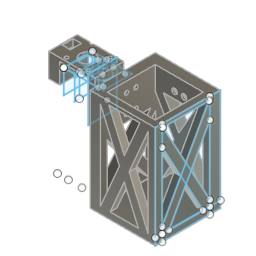
Chocolate_Extruder_v12_v4 (Autodesk Fusion 360 design; units mm, degrees)
Autodesk Fusion 360 part; units mm, degrees
note: some values were not read from the file. Chosen so that the rebuilt part matches the saved one: which pieces of a blend or face edit are solid. Set by a fixed rule: which sketch regions a step uses.
sketch "Sketch1" plane through (0, 0, 0) normal (0, 0, 1) x (1, 0, 0)
  line L0 (0, 70.5) -> (70.5, 70.5)
  line L1 (70.5, 70.5) -> (70.5, 0)
  line L2 (70.5, 0) -> (0, 0)
  line L3 (0, 0) -> (0, 70.5)
  line L4 (-15, 85.5) -> (75.5, 85.5)
  line L5 (75.5, 85.5) -> (75.5, -5)
  line L6 (75.5, -5) -> (-15, -5)
  line L7 (-15, -5) -> (-15, 85.5)
  circle A0 centre (35.25, 35.25) radius 5.5
  dimension "d1" = 70.5
  dimension "d2" = 70.5
  dimension "d3" = 5
  dimension "d4" = 5
  dimension "d5" = 15
  dimension "d6" = 15
  dimension "d9" = 11
  dimension "d10" = 35.25
  dimension "d11" = 35.25
  constraint horizontal L0
  constraint vertical L1
  constraint horizontal L2
  constraint vertical L3
  constraint coincident L2.end L3.start
  constraint horizontal L4
  constraint vertical L5
  constraint horizontal L6
  constraint vertical L7
  measures "d1" distance of L1 L3
  measures "d2" distance of L0 L2
  measures "d3" distance of L1 L5
  measures "d4" distance of L2 L6
  measures "d5" distance of L0 L4
  measures "d6" distance of L3 L7
  measures "d9" diameter of A0
  measures "d10" distance of L3 A0.centre
  measures "d11" distance of L0 A0.centre
extrude "Extrude1" add sketch "Sketch1" along normal blind 140 contours L4 L5 L6 L7 makes body 1
extrude "Extrude2" add sketch "Sketch1" against normal blind 10 contours L0 L1 L2 L3 | L4 L5 L6 L7 bodies 1
sketch "Sketch2" plane through (0, 0, -10) normal (0, 0, -1) x (1, 0, 0)
  circle A0 centre (35.25, -35.25) radius 5.5
  line L0 (75.5, 5) -> (-15, 5)
  line L1 (-15, 5) -> (-15, -85.5)
  line L2 (-15, -85.5) -> (75.5, -85.5)
  line L3 (75.5, -85.5) -> (75.5, 5)
ref_plane "WorkPlane1" through (35.25, 35.25, 125) normal (0, 0, -1) x (1, 0, 0)
sketch "Sketch3" plane through (0, 0, 125) normal (0, 0, -1) x (-1, 0, 0)
  line L0 (15, 14.25) -> (57, 14.25)
  line L1 (57, 14.25) -> (57, 56.25)
  line L2 (57, 56.25) -> (15, 56.25)
  line L3 (15, 56.25) -> (15, 14.25)
  circle A0 centre (36, 34.25) radius 11
  circle A1 centre (36, 34.25) radius 16
  circle A2 centre (20, 19.25) radius 2.5
  circle A3 centre (20, 51.25) radius 2.2361
  line L4 (15, -5) -> (15, 85.5)
  circle A4 centre (52, 19.25) radius 2.5
  circle A5 centre (52, 51.25) radius 2.2361
  dimension "d15" = 21
  dimension "d16" = 20
  dimension "d17" = 22
  dimension "d18" = 42
  dimension "d19" = 22
  dimension "d20" = 5
  dimension "d21" = 5
  dimension "d22" = 5
  dimension "d23" = 5
  dimension "d24" = 5
  dimension "d26" = 42
  dimension "d27" = 19.25
  dimension "d28" = 29.25
  dimension "d29" = 5
  dimension "d30" = 5
  constraint horizontal L0
  constraint vertical L1
  constraint vertical L3
  constraint coincident L2.end L4
  measures "d15" distance of L3 A0.centre
  measures "d16" distance of L0 A0.centre
  measures "d17" distance of L2 A0.centre
  measures "d18" distance of L0 L2
  measures "d19" diameter of A0
  measures "d21" distance of L0 A2.centre
  measures "d22" distance of L3 A2.centre
  measures "d23" diameter of A2
  measures "d24" distance of L3 A3.centre
  measures "d26" distance of L1 L3
  measures "d27" distance of L0 L4.start
  measures "d28" distance of L2.end L4.end
  measures "d29" diameter of A4
  measures "d30" distance of L0 A4.centre
extrude "Extrude3" add sketch "Sketch3" against normal blind 5 separate body contours L0 L1 L2 L3 L4 | A1 makes body 2
sketch "Sketch4" plane through (0, 0, 130) normal (0, 0, 1) x (-1, 0, 0)
  circle A0 centre (36, -34.25) radius 11
  circle A1 centre (20, -51.25) radius 2.2361
  circle A2 centre (20, -19.25) radius 2.5
  circle A3 centre (52, -19.25) radius 2.5
  line L0 (15, -14.25) -> (15, -56.25)
  line L1 (15, -56.25) -> (57, -56.25)
  line L2 (57, -56.25) -> (57, -14.25)
  circle A4 centre (36, -34.25) radius 6
  line L3 (36, -34.25) -> (57, -34.25)
  line L4 (36, -34.25) -> (15, -34.25)
  circle A5 centre (52, -51.25) radius 2.2361
  dimension "d36" = 12
  constraint concentric A0 A4
  constraint coincident A0.centre A4.centre
  constraint coincident L2 L3.end
  constraint perpendicular L2 L3
  constraint coincident L0 L4.end
  constraint perpendicular L0 L4
  measures "d36" diameter of A4
ref_plane "WorkPlane2" through (-36, 34.25, 127.5) normal (0, -1, 0) x (1, 0, 0)
sketch "Sketch5" plane through (0, 34.25, 0) normal (0, -1, 0) x (-1, 0, 0)
  line L0 (30, -130) -> (42, -130)
  line L1 (42, -130) -> (42, -150)
  line L2 (42, -150) -> (30, -150)
  line L3 (30, -150) -> (30, -130)
  line L4 (42.8404, -129.1596) -> (42.8404, -150.8404)
  line L5 (42.8404, -150.8404) -> (29.1596, -150.8404)
  line L6 (29.1596, -150.8404) -> (29.1596, -129.1596)
  line L7 (29.1596, -129.1596) -> (42.8404, -129.1596)
  line L8 (30, -130) -> (29.1596, -130)
  line L9 (29.1596, -130) -> (42, -130)
  line L10 (42.8404, -130) -> (42, -130)
  line L11 (52.8404, -130) -> (42.8404, -140)
  line L12 (36, -130) -> (57, -130)
  line L13 (29.1596, -140) -> (19.1596, -130)
  line L14 (36, -130) -> (15, -130)
  line L15 (24.1596, -130) -> (29.1596, -135)
  line L16 (47.8404, -130) -> (42.8404, -135)
  line L17 (36, -150) -> (36, -150.8404)
  line L18 (42.8404, -135) -> (42, -135.8404)
  line L19 (29.1596, -135) -> (30, -135.8404)
  line L20 (42, -150) -> (42.8404, -150)
  point P0 (36, -130)
  point P1 (36, -150)
  dimension "d38" = 6
  dimension "d39" = 6
  dimension "d40" = -0.8404
  dimension "d41" = 20
  dimension "d42" = 10
  dimension "d43" = 10
  dimension "d44" = 10
  dimension "d45" = 10
  dimension "d46" = 5
  dimension "d47" = 5
  dimension "d48" = 5
  dimension "d49" = 5
  constraint horizontal L0
  constraint vertical L1
  constraint horizontal L2
  constraint vertical L3
  constraint coincident L0 P0
  constraint coincident L6 L8.end
  constraint perpendicular L6 L8
  constraint coincident L4 L10.start
  constraint perpendicular L1 L10
  constraint coincident L4 L11.end
  constraint coincident L11.start L12
  constraint coincident L6 L13.start
  constraint coincident L13.end L14
  constraint midpoint L2 P1
  constraint coincident L14 L15.start
  constraint coincident L6 L15.end
  constraint coincident L12 L16.start
  constraint coincident L4 L16.end
  constraint coincident P1 L17.start
  constraint midpoint L5 L17.end
  constraint coincident L1 L18.end
  constraint parallel L16 L18
  constraint coincident L3 L19.end
  constraint perpendicular L18 L19
  constraint coincident L4 L20.end
  constraint perpendicular L4 L20
  measures "d38" distance of L1 P0
  measures "d39" distance of L3 P0
  measures "d41" distance of L0 L2
  measures "d42" distance of L10.start L11.end
  measures "d43" distance of L10.start L11.start
  measures "d44" distance of L8.end L13.end
  measures "d45" distance of L8.end L13.start
  measures "d46" distance of L6 L15.start
  measures "d47" distance of L8.end L15.end
  measures "d48" distance of L10.start L16.start
  measures "d49" distance of L10.start L16.end
revolve "Revolve1" [suppressed]
sketch "Sketch6" plane through (-57, 0, 0) normal (-1, 0, 0) x (0, -1, 0)
  line L0 (-56.25, 125) -> (-14.25, 125)
  line L1 (-14.25, 125) -> (-14.25, 130)
  line L2 (-14.25, 130) -> (-56.25, 130)
  line L3 (-56.25, 130) -> (-56.25, 125)
  line L4 (-56.25, 130) -> (-14.25, 130)
  line L5 (-14.25, 130) -> (-14.25, 95)
  line L6 (-14.25, 95) -> (-56.25, 95)
  line L7 (-56.25, 95) -> (-56.25, 130)
  line L8 (-49.25, 130) -> (-49.25, 95)
  line L9 (-21.25, 130) -> (-21.25, 95)
  dimension "d51" = 30
  dimension "d151" = 7
  dimension "d152" = 7
  constraint horizontal L4
  constraint vertical L5
  constraint horizontal L6
  constraint vertical L7
  constraint coincident L2.end L3.start
  constraint coincident L0.end L5
  constraint coincident L4 L8.start
  constraint coincident L6 L8.end
  constraint perpendicular L6 L8
  constraint coincident L4 L9.start
  constraint coincident L6 L9.end
  constraint perpendicular L6 L9
  measures "d51" distance of L0 L6
  measures "d151" distance of L7 L8
  measures "d152" distance of L5 L9
extrude "Extrude4" add sketch "Sketch6" along normal blind 16 bodies 2
sketch "Sketch7" plane through (-73, 0, 0) normal (-1, 0, 0) x (0, -1, 0)
  line L0 (-56.25, 95) -> (-14.25, 95)
  line L1 (-14.25, 130) -> (-56.25, 130)
  line L2 (-14.25, 95) -> (-14.25, 130)
  line L3 (-56.25, 130) -> (-56.25, 95)
sketch "Sketch8" plane through (0, 0, 130) normal (0, 0, 1) x (-1, 0, 0)
  circle A0 centre (20, -51.25) radius 2.2361
  circle A1 centre (52, -19.25) radius 2.5
  circle A2 centre (20, -19.25) radius 2.5
  line L0 (73, -14.25) -> (15, -14.25)
  line L1 (15, -14.25) -> (15, -56.25)
  line L2 (15, -56.25) -> (73, -56.25)
  line L3 (73, -56.25) -> (73, -14.25)
  line L4 (59, -27) -> (71, -27)
  line L5 (71, -27) -> (71, -43)
  line L6 (71, -43) -> (59, -43)
  line L7 (59, -43) -> (59, -27)
  line L8 (73, -14.25) -> (73, -56.25)
  circle A3 centre (36, -34.25) radius 11
  circle A4 centre (52, -51.25) radius 2.2361
  dimension "d54" = 2
  dimension "d55" = 16
  dimension "d56" = 12
  constraint horizontal L4
  constraint vertical L5
  constraint horizontal L6
  constraint vertical L7
  measures "d54" distance of L5 L8
  measures "d55" distance of L4 L6
  measures "d56" distance of L5 L7
extrude "Extrude5" cut sketch "Sketch8" against normal blind 10 contours L4 L5 L6 L7 bodies 2
sketch "Sketch11" plane through (0, 70.5, 0) normal (0, -1, 0) x (1, 0, 0)
  line L0 (0, 0) -> (70.5, 0)
  line L1 (70.5, 0) -> (70.5, 140)
  line L2 (70.5, 140) -> (0, 140)
  line L3 (0, 140) -> (0, 0)
  circle A0 centre (28.25, 120) radius 4
  circle A1 centre (42.25, 120) radius 4
  circle A2 centre (28.25, 120) radius 2
  circle A3 centre (42.25, 120) radius 2
  line L4 (0, 0) -> (70.5, 0)
  dimension "d77" = 8
  dimension "d78" = 28.25
  dimension "d79" = 14
  dimension "d80" = 8
  dimension "d83" = 4
  dimension "d84" = 4
  dimension "d87" = 120
  constraint concentric A0 A2
  constraint concentric A1 A3
  measures "d77" diameter of A0
  measures "d78" distance of L1 A1.centre
  measures "d79" distance of A0.centre A1.centre
  measures "d80" diameter of A1
  measures "d83" diameter of A2
  measures "d84" diameter of A3
  measures "d87" distance of A1.centre L4
extrude "Extrude8" cut sketch "Sketch11" against normal blind 3 contours A0 | A1 | A2 | A3 bodies 1
extrude "Extrude9" cut sketch "Sketch11" against normal blind 15 contours A2 | A3 bodies 1
move_body "Move1" bodies 2 to x (1, 0, 0) y (0, 1, 0) z (0, 0, 1) at (-22.0189, -0.0781, 10)
sketch "Sketch12" plane through (-37.0189, 0, 0) normal (1, 0, 0) x (0, 1, 0)
  line L0 (14.1719, 135) -> (56.1719, 135)
  line L1 (56.1719, 135) -> (56.1719, 140)
  line L2 (56.1719, 140) -> (14.1719, 140)
  line L3 (14.1719, 140) -> (14.1719, 135)
  line L4 (14.1719, 140) -> (56.1719, 140)
  line L5 (56.1719, 140) -> (56.1719, 75)
  line L6 (56.1719, 75) -> (14.1719, 75)
  line L7 (14.1719, 75) -> (14.1719, 140)
  point P0 (51.25, 130)
  dimension "d88" = 42
  dimension "d93" = 60
  constraint horizontal L4
  constraint vertical L5
  constraint horizontal L6
  constraint vertical L7
  constraint coincident L2.end L3.start
  measures "d88" distance of L5 L7
  measures "d93" distance of L0 L6
extrude "Extrude10" add sketch "Sketch12" along normal blind 10 bodies 2
sketch "Sketch16" plane through (0, 0, 0) normal (1, 0, 0) x (0, 1, 0)
  line L0 (0, 0) -> (70.5, 0)
  line L1 (70.5, 0) -> (70.5, 140)
  line L2 (70.5, 140) -> (0, 140)
  line L3 (0, 140) -> (0, 0)
  line L4 (0, 125) -> (70.5, 125)
  line L5 (0, 98) -> (70.5, 98)
  circle A0 centre (28.25, 125) radius 2
  circle A1 centre (42.25, 125) radius 2
  circle A2 centre (28.25, 98) radius 2
  circle A3 centre (42.25, 98) radius 2
  line L6 (70.5, 140) -> (70.5, 0)
  circle A4 centre (42.25, 125) radius 3
  circle A5 centre (28.25, 125) radius 3
  circle A6 centre (28.25, 98) radius 3
  circle A7 centre (42.25, 98) radius 3
  point P0 (35.25, 140)
  dimension "d121" = 4
  dimension "d122" = 4
  dimension "d123" = 4
  dimension "d124" = 4
  dimension "d125" = 14
  dimension "d126" = 14
  dimension "d127" = 28.25
  dimension "d128" = 28.25
  dimension "d129" = 28.25
  dimension "d130" = 28.25
  dimension "d131" = 1
  dimension "d132" = 1
  dimension "d133" = 1
  dimension "d134" = 1
  dimension "d137" = 15
  dimension "d138" = 27
  constraint coincident L3 L4.start
  constraint coincident L1 L4.end
  constraint perpendicular L1 L4
  constraint coincident L3 L5.start
  constraint coincident L1 L5.end
  constraint perpendicular L1 L5
  constraint coincident L4 A0.centre
  constraint coincident L4 A1.centre
  constraint coincident L5 A2.centre
  constraint coincident L5 A3.centre
  constraint midpoint L2 P0
  measures "d121" diameter of A0
  measures "d122" diameter of A1
  measures "d123" diameter of A2
  measures "d124" diameter of A3
  measures "d125" distance of A0.centre A1.centre
  measures "d126" distance of A2.centre A3.centre
  measures "d127" distance of A1.centre L6
  measures "d128" distance of L3 A0.centre
  measures "d129" distance of L3 A2.centre
  measures "d130" distance of A3.centre L6
  measures "d137" distance of L2 L4
  measures "d138" distance of L4 L5
extrude "Extrude14" cut sketch "Sketch16" against normal blind 37.019 contours L5 A2 | L5 A2 | L5 A3 | L5 A3 | L4 A0 | L4 A0 | L4 A1 | L4 A1 bodies 1 2
extrude "Extrude15" cut sketch "Sketch16" against normal blind 3 contours L5 A2 A6 | L5 A2 A6 | L5 A3 A7 | L5 A3 A7 | L4 A0 A5 | L4 A0 A5 | L5 A2 | L5 A2 | L4 A1 A4 | L4 A1 A4 | L5 A3 | L5 A3 | L4 A0 | L4 A0 | L4 A1 | L4 A1 bodies 1
sketch "Sketch21" plane through (75.5, 0, 0) normal (1, 0, 0) x (0, 1, 0)
  line L0 (85.5, -10) -> (85.5, 140)
  line L1 (85.5, 140) -> (-5, 140)
  line L2 (-5, 140) -> (-5, -10)
  line L3 (-5, -10) -> (85.5, -10)
  line L4 (0, 0) -> (0, -10)
  line L5 (0, 0) -> (0, 140)
  line L6 (70, 140) -> (70, -10)
  line L7 (0, 135) -> (70, 135)
  line L8 (0, 0) -> (70, 0)
  line L9 (0, 110) -> (60, 0)
  line L10 (1.1565, 135) -> (70, 8.787)
  line L11 (10, 0) -> (70, 110)
  line L12 (68.5277, 135) -> (0, 9.366)
  line L13 (85.5, 0) -> (-5, 0)
  dimension "d149" = 5
  dimension "d150" = 10
  constraint coincident L4.start L5.start
  constraint coincident L3 L4.end
  constraint perpendicular L3 L4
  constraint coincident L1 L5.end
  constraint perpendicular L1 L5
  constraint coincident L1 L6.start
  constraint coincident L3 L6.end
  constraint perpendicular L3 L6
  constraint coincident L5 L7.start
  constraint coincident L6 L7.end
  constraint perpendicular L6 L7
  constraint coincident L6 L8.end
  constraint perpendicular L6 L8
  constraint coincident L5 L9.start
  constraint coincident L8 L9.end
  constraint coincident L7 L10.start
  constraint coincident L6 L10.end
  constraint parallel L9 L10
  constraint coincident L8 L11.start
  constraint coincident L6 L11.end
  constraint coincident L7 L12.start
  constraint coincident L5 L12.end
  constraint parallel L11 L12
  measures "d149" distance of L1 L7
  measures "d150" distance of L3 L13
extrude "Extrude18" cut sketch "Sketch21" against normal blind 10 contours L6 L10 L11 | L8 L9 L11 L13 | L5 L9 L12 | L7 L10 L12 bodies 1
sketch "Sketch22" plane through (0, -5, 0) normal (0, -1, 0) x (1, 0, 0)
  line L0 (75.5, -10) -> (75.5, 140)
  line L1 (75.5, 140) -> (-15, 140)
  line L2 (-15, 140) -> (-15, -10)
  line L3 (-15, -10) -> (75.5, -10)
  line L4 (0, 140) -> (0, -10)
  line L5 (70, 140) -> (70, -10)
  line L6 (60, -10) -> (0, 130)
  line L7 (10, -10) -> (70, 130)
  line L8 (60, 140) -> (0, 0)
  line L9 (10, 140) -> (70, 0)
  line L10 (-15, 0) -> (75.5, 0)
  line L11 (75.5, 134.8901) -> (-15, 134.8901)
  constraint coincident L1 L4.start
  constraint coincident L3 L4.end
  constraint perpendicular L3 L4
  constraint coincident L1 L5.start
  constraint coincident L3 L5.end
  constraint perpendicular L3 L5
  constraint coincident L3 L6.start
  constraint coincident L4 L6.end
  constraint coincident L3 L7.start
  constraint coincident L5 L7.end
  constraint coincident L1 L8.start
  constraint coincident L8.end origin
  constraint parallel L7 L8
  constraint coincident L1 L9.start
  constraint coincident L5 L9.end
  constraint parallel L6 L9
  constraint coincident L2 L10.start
  constraint coincident L0 L10.end
  constraint perpendicular L0 L10
  constraint coincident L0 L11.start
  constraint coincident L2 L11.end
  constraint perpendicular L2 L11
extrude "Extrude19" cut sketch "Sketch22" against normal blind 10 contours L5 L7 L9 | L6 L7 L10 | L8 L9 L11 | L4 L6 L8 bodies 1
sketch "Sketch23" plane through (0, 85.5, 0) normal (0, 1, 0) x (-1, 0, 0)
  circle A0 centre (-42.25, 120) radius 2
  circle A1 centre (-28.25, 120) radius 2
  line L0 (15, -10) -> (15, 140)
  line L1 (15, 140) -> (-75.5, 140)
  line L2 (-75.5, 140) -> (-75.5, -10)
  line L3 (-75.5, -10) -> (15, -10)
  line L4 (-70, 140) -> (-70, -10)
  line L5 (0, 140) -> (0, -10)
  line L6 (-75.5, 0) -> (15, 0)
  line L7 (-75.5, 110) -> (15, 110)
  line L8 (-70, 110) -> (-10, 0)
  line L9 (0, 10) -> (-57.4408, 110)
  line L10 (-60.3129, 0) -> (0, 105.9676)
  line L11 (-11.909, 110) -> (-70, 7.9362)
  dimension "d155" = 10
  constraint coincident L1 L4.start
  constraint coincident L3 L4.end
  constraint perpendicular L3 L4
  constraint coincident L1 L5.start
  constraint coincident L3 L5.end
  constraint perpendicular L3 L5
  constraint coincident L2 L6.start
  constraint coincident L0 L6.end
  constraint perpendicular L0 L6
  constraint coincident L2 L7.start
  constraint coincident L0 L7.end
  constraint perpendicular L0 L7
  constraint coincident L4 L8.start
  constraint coincident L6 L8.end
  constraint coincident L5 L9.start
  constraint coincident L7 L9.end
  constraint coincident L6 L10.start
  constraint coincident L5 L10.end
  constraint coincident L7 L11.start
  constraint coincident L4 L11.end
  constraint parallel L10 L11
  measures "d155" distance of A0.centre L7
extrude "Extrude20" cut sketch "Sketch23" against normal blind 15 contours L5 L9 L10 | L6 L8 L10 | L7 L9 L11 | L4 L8 L11 bodies 1
sketch "Sketch24" plane through (-15, 0, 0) normal (-1, 0, 0) x (0, -1, 0)
  circle A0 centre (-42.25, 125) radius 2
  circle A1 centre (-42.25, 98) radius 2
  circle A2 centre (-28.25, 125) radius 2
  circle A3 centre (-28.25, 98) radius 2
  line L0 (5, -10) -> (5, 140)
  line L1 (5, 140) -> (-85.5, 140)
  line L2 (-85.5, 140) -> (-85.5, -10)
  line L3 (-85.5, -10) -> (5, -10)
  line L4 (-85.5, 88) -> (5, 88)
  line L5 (-85.5, 0.6227) -> (5, 0.6227)
  line L6 (0.0167, 140) -> (0.0167, -10)
  line L7 (-70.8768, 140) -> (-70.8768, -10)
  line L8 (-70.8768, 80.9133) -> (-9.5001, 0.6227)
  line L9 (-63.7873, 88) -> (0.0167, 10.341)
  line L10 (-61.9234, 0.6227) -> (0.0167, 79.5561)
  line L11 (-9.5001, 88) -> (-70.8768, 9.7847)
  dimension "d158" = 10
  constraint coincident L2 L4.start
  constraint coincident L0 L4.end
  constraint perpendicular L0 L4
  constraint coincident L2 L5.start
  constraint coincident L0 L5.end
  constraint perpendicular L0 L5
  constraint coincident L1 L6.start
  constraint coincident L3 L6.end
  constraint perpendicular L3 L6
  constraint coincident L1 L7.start
  constraint coincident L3 L7.end
  constraint perpendicular L3 L7
  constraint coincident L7 L8.start
  constraint coincident L5 L8.end
  constraint coincident L4 L9.start
  constraint coincident L6 L9.end
  constraint coincident L5 L10.start
  constraint coincident L6 L10.end
  constraint coincident L4 L11.start
  constraint coincident L7 L11.end
  constraint parallel L10 L11
  measures "d158" distance of A3.centre L4
extrude "Extrude21" cut sketch "Sketch24" against normal blind 15 contours L5 L8 L10 | L6 L9 L10 | L4 L9 L11 | L7 L8 L11 bodies 1
copy_body "Body->Comp1" bodies 1 removing the originals makes body 3 in component "Component"
copy_body "Body->Comp2" bodies 2 removing the originals makes body 4 in component "Component'"
fillet "Fillet1" radius 5 48 edges at (57.4408, 78, 110) (11.909, 78, 110) (35, -2.5, 81.6667) (42.1429, -2.5, 65) (27.8571, -2.5, 65) (35, -2.5, 48.3333) (34.5705, 78, 70.1846) (27.4359, 78, 57.7637) (41.5723, 78, 57.8826) (34.6213, 78, 45.1391) (10, 78, 0) (60.3129, 78, 0) (0, 78.1884, 10) (-7.5, 70.8768, 9.7847) (70, 78, 7.9362) (73, 70, 8.787) (73, 60, 0) (73, 10, 0) (70, -2.5, 0) (73, 0, 9.366) (0, -2.5, 0) (14.2857, -2.5, 0) (55.7143, -2.5, 0) (73, 42.3964, 59.3935) (73, 27.4456, 59.683) (73, 34.8421, 73.2431) (73, 35, 45.8333) (73, 1.1565, 135) (73, 68.5277, 135) (12.19, -2.5, 134.8901) (57.81, -2.5, 134.8901) (0, -2.5, 130) (70, -2.5, 130) (73, 70, 110) (73, 0, 110) (70, 78, 110) (0, 78, 105.9676) (-7.5, 61.9234, 0.6227) (-7.5, 9.5001, 0.6227) (-7.5, -0.0167, 10.341) (-7.5, 27.7638, 44.154) (-7.5, 35.3686, 34.4628) (-7.5, 43.3344, 44.8834) (-7.5, 36.0206, 54.2037) (-7.5, 9.5001, 88) (-7.5, 63.7873, 88) (-7.5, -0.0167, 79.5561) (-7.5, 70.8768, 80.9133) on bodies 3 in component "Component"
sketch "Sketch25" plane through (0, 85.5, 0) normal (0, 1, 0) x (-1, 0, 0)
  line L0 (-30.3248, 37.2621) -> (-14.0332, 7.3943)
  arc A0 (-18.4227, 0) -> (-14.0332, 7.3943) centre (-18.4227, 5) ccw
  line L1 (-18.4227, 0) -> (-51.7139, 0)
  arc A1 (-56.0594, 7.4733) -> (-51.7139, 0) centre (-51.7139, 5) ccw
  line L2 (-56.0594, 7.4733) -> (-39.0597, 37.3411)
  arc A2 (-30.3248, 37.2621) -> (-39.0597, 37.3411) centre (-34.7143, 34.8678) ccw
  line L3 (-42.9506, 55.4611) -> (-60.6546, 24.3558)
  arc A3 (-70, 26.8291) -> (-60.6546, 24.3558) centre (-65, 26.8291) ccw
  line L4 (-70, 26.8291) -> (-70, 90.3917)
  arc A4 (-60.6105, 92.786) -> (-70, 90.3917) centre (-65, 90.3917) ccw
  line L5 (-60.6105, 92.786) -> (-42.9065, 60.3287)
  arc A5 (-42.9506, 55.4611) -> (-42.9065, 60.3287) centre (-47.296, 57.9344) ccw
  line L6 (-26.0217, 60.2484) -> (-9.3454, 89.548)
  arc A6 (0, 87.0747) -> (-9.3454, 89.548) centre (-5, 87.0747) ccw
  line L7 (0, 87.0747) -> (0, 28.743)
  arc A7 (-9.3356, 26.2526) -> (0, 28.743) centre (-5, 28.743) ccw
  line L8 (-9.3356, 26.2526) -> (-26.0119, 55.2847)
  arc A8 (-26.0217, 60.2484) -> (-26.0119, 55.2847) centre (-21.6763, 57.7751) ccw
  line L9 (-38.9261, 77.7672) -> (-53.1383, 102.5096)
  arc A9 (-48.8026, 110) -> (-53.1383, 102.5096) centre (-48.8026, 105) ccw
  line L10 (-48.8026, 110) -> (-20.508, 110)
  arc A10 (-16.1626, 102.5267) -> (-20.508, 110) centre (-20.508, 105) ccw
  line L11 (-16.1626, 102.5267) -> (-30.245, 77.7844)
  arc A11 (-38.9261, 77.7672) -> (-30.245, 77.7844) centre (-34.5904, 80.2577) ccw
  circle A12 centre (-42.25, 120) radius 2
  circle A13 centre (-28.25, 120) radius 2
  line L12 (15, -10) -> (15, 140)
  line L13 (15, 140) -> (-75.5, 140)
  line L14 (-75.5, 140) -> (-75.5, -10)
  line L15 (-75.5, -10) -> (15, -10)
  circle A14 centre (-42.25, 120) radius 2
  circle A15 centre (-28.25, 120) radius 2
  line L16 (-42.25, 110) -> (-28.25, 110)
  arc A16 (-28.25, 110) -> (-28.25, 130) centre (-28.25, 120) ccw
  line L17 (-28.25, 130) -> (-42.25, 130)
  arc A17 (-42.25, 130) -> (-42.25, 110) centre (-42.25, 120) ccw
  line L18 (-42.25, 120) -> (-28.25, 120) construction
  dimension "d163" = 20
  constraint tangent L16 A16
  constraint tangent A16 L17
  constraint parallel L16 L17
  constraint tangent L17 A17
  constraint tangent L16 A17
  constraint coincident A13.centre A15.centre
  constraint coincident A12.centre A14.centre
  measures "d163" diameter of A16
extrude "Extrude1'" cut sketch "Sketch25" against normal blind 10 contours L12 L13 L14 L15 bodies 3 in component "Component"
sketch "Sketch1 (2)" plane through (-15, 0, 0) normal (-1, 0, 0) x (0, -1, 0) in component "Component"
  line L0 (-75.5, 140) -> (-75.5, -10)
  line L1 (-75.5, -10) -> (5, -10)
  line L2 (5, -10) -> (5, 140)
  line L3 (5, 140) -> (-75.5, 140)
  circle A0 centre (-28.25, 98) radius 2
  circle A1 centre (-28.25, 125) radius 2
  circle A2 centre (-42.25, 98) radius 2
  circle A3 centre (-42.25, 125) radius 2
  line L4 (-8.8466, 21.1289) -> (-25.215, 41.0518)
  arc A4 (-25.2852, 47.3125) -> (-25.215, 41.0518) centre (-21.3517, 44.2259) ccw
  line L5 (-25.2852, 47.3125) -> (-8.9168, 68.1717)
  arc A5 (0.0167, 65.085) -> (-8.9168, 68.1717) centre (-4.9833, 65.085) ccw
  line L6 (0.0167, 65.085) -> (0.0167, 24.303)
  arc A6 (-8.8466, 21.1289) -> (0.0167, 24.303) centre (-4.9833, 24.303) ccw
  line L7 (-31.448, 29.3341) -> (-15.6435, 8.6593)
  arc A7 (-19.6158, 0.6227) -> (-15.6435, 8.6593) centre (-19.6158, 5.6227) ccw
  line L8 (-19.6158, 0.6227) -> (-51.6441, 0.6227)
  arc A8 (-55.5776, 8.7094) -> (-51.6441, 0.6227) centre (-51.6441, 5.6227) ccw
  line L9 (-55.5776, 8.7094) -> (-39.3538, 29.3842)
  arc A9 (-31.448, 29.3341) -> (-39.3538, 29.3842) centre (-35.4203, 26.2975) ccw
  line L10 (-15.8459, 79.9133) -> (-32.1766, 59.1023)
  arc A10 (-39.9734, 59.0149) -> (-32.1766, 59.1023) centre (-36.1101, 62.189) ccw
  line L11 (-39.9734, 59.0149) -> (-57.0716, 79.8259)
  arc A11 (-53.2082, 88) -> (-57.0716, 79.8259) centre (-53.2082, 83) ccw
  line L12 (-53.2082, 88) -> (-19.7794, 88)
  arc A12 (-15.8459, 79.9133) -> (-19.7794, 88) centre (-19.7794, 83) ccw
  line L13 (-45.7251, 41.8368) -> (-61.9433, 21.1691)
  arc A13 (-70.8768, 24.2557) -> (-61.9433, 21.1691) centre (-65.8768, 24.2557) ccw
  line L14 (-70.8768, 24.2557) -> (-70.8768, 66.1395)
  arc A14 (-61.9045, 69.176) -> (-70.8768, 66.1395) centre (-65.8768, 66.1395) ccw
  line L15 (-61.9045, 69.176) -> (-45.6863, 47.96)
  arc A15 (-45.7251, 41.8368) -> (-45.6863, 47.96) centre (-49.6586, 44.9234) ccw
  circle A16 centre (-28.25, 125) radius 2
  circle A17 centre (-42.25, 125) radius 2
  circle A18 centre (-42.25, 98) radius 2
  circle A19 centre (-28.25, 98) radius 2
  line L16 (-28.25, 125) -> (-42.25, 98) construction
  line L17 (-43.25, 130) -> (-27.25, 130)
  line L18 (-23.25, 126) -> (-23.25, 97)
  line L19 (-27.25, 93) -> (-43.25, 93)
  line L20 (-47.25, 97) -> (-47.25, 126)
  line L21 (-47.25, 130) -> (-23.25, 93) construction
  line L22 (-23.25, 130) -> (-47.25, 93) construction
  arc A20 (-43.25, 130) -> (-47.25, 126) centre (-43.25, 126) ccw
  arc A21 (-47.25, 97) -> (-43.25, 93) centre (-43.25, 97) ccw
  arc A22 (-27.25, 93) -> (-23.25, 97) centre (-27.25, 97) ccw
  arc A23 (-23.25, 126) -> (-27.25, 130) centre (-27.25, 126) ccw
  point P0 (-35.25, 111.5)
  point P1 (-35.25, 111.5)
  dimension "d166" = 5
  dimension "d167" = 5
  dimension "d168" = 4
  dimension "d169" = 4
  constraint coincident A1.centre A16.centre
  constraint coincident A2.centre A18.centre
  constraint midpoint L16 P1
  constraint horizontal L17
  constraint perpendicular L17 L18
  constraint parallel L17 L19
  constraint parallel L18 L20
  constraint coincident L21 P1
  constraint coincident L22 P1
  constraint coincident P1 P0
  constraint coincident L21.start L17
  constraint coincident L21.start L20
  constraint tangent L17 A20
  constraint tangent L20 A20
  constraint coincident L22.end L19
  constraint coincident L22.end L20
  constraint tangent L19 A21
  constraint tangent L20 A21
  constraint equal A20 A21
  constraint coincident L21.end L19
  constraint coincident L21.end L18
  constraint tangent L19 A22
  constraint tangent L18 A22
  constraint equal A20 A22
  constraint coincident L22.start L17
  constraint coincident L22.start L18
  constraint tangent L17 A23
  constraint tangent L18 A23
  measures "d166" distance of A3.centre L17
  measures "d167" distance of A3.centre L20
  measures "d168" radius of A20
  measures "d169" radius of A23
extrude "Extrude2'" cut sketch "Sketch1 (2)" against normal blind 10 contours L0 L1 L2 L3 bodies 3 in component "Component"
extrude "Extrude3'" cut 1 faces at (35.387, 6.5885, -10) along direction (0, 0, 1) blind 5 on bodies 3 bodies 3 in component "Component"
sketch "Sketch1 (3)" plane through (-27.0189, 0, 0) normal (1, 0, 0) x (0, 1, 0) in component "Component'"
  circle A0 centre (42.25, 125) radius 2
  circle A1 centre (42.25, 98) radius 2
  circle A2 centre (28.25, 125) radius 2
  circle A3 centre (28.25, 98) radius 2
  line L0 (14.1719, 75) -> (56.1719, 75)
  line L1 (56.1719, 75) -> (56.1719, 140)
  line L2 (56.1719, 140) -> (14.1719, 140)
  line L3 (14.1719, 140) -> (14.1719, 75)
  line L4 (43.25, 93) -> (27.25, 93)
  arc A4 (23.25, 97) -> (27.25, 93) centre (27.25, 97) ccw
  line L5 (23.25, 97) -> (23.25, 126)
  arc A5 (27.25, 130) -> (23.25, 126) centre (27.25, 126) ccw
  line L6 (27.25, 130) -> (43.25, 130)
  arc A6 (47.25, 126) -> (43.25, 130) centre (43.25, 126) ccw
  line L7 (47.25, 126) -> (47.25, 97)
  arc A7 (43.25, 93) -> (47.25, 97) centre (43.25, 97) ccw
  circle A8 centre (28.25, 98) radius 2
  circle A9 centre (28.25, 125) radius 2
  circle A10 centre (42.25, 98) radius 2
  circle A11 centre (42.25, 125) radius 2
  line L8 (23.3347, 96.1813) -> (14.1719, 140)
  line L9 (47.1681, 96.1947) -> (56.1719, 140)
  constraint coincident A4 L8.start
  constraint coincident L2.end L3.start
  constraint coincident A7 L9.start
  constraint coincident L1.end L2.start
  constraint tangent A7 L9
  constraint tangent A4 L8
extrude "Extrude1''" cut sketch "Sketch1 (3)" against normal blind 68 contours L0 L1 L3 L4 A4 A7 L8 L9 bodies 4 in component "Component'"
fillet "Fillet1'" radius 5 2 edges at (-87.0189, 48.9779, 105) (-87.0189, 21.4906, 105) on bodies 4 in component "Component'"
extrude "Extrude3''" cut 1 faces at (-85.0189, 32.2552, 130) along direction (0, 0, -1) blind 20 on bodies 4 bodies 4 in component "Component'"
fillet "Fillet2" radius 0.5 4 edges at (-61.0189, 14.1719, 140) (-95.0189, 35.1719, 140) (-61.0189, 56.1719, 140) (-27.0189, 35.1719, 140) on bodies 4 in component "Component'"
fillet "Fillet3" radius 0.5 4 edges at (-81.0189, 34.9219, 140) (-87.0189, 42.9219, 140) (-93.0189, 34.9219, 140) (-87.0189, 26.9219, 140) on bodies 4 in component "Component'"
component "Component" placed x (1, 0, 0) y (0, 1, 0) z (0, 0, 1) at (0, 0, 0)
component "Component'" placed x (1, 0, 0) y (0, 1, 0) z (0, 0, 1) at (0, 0, 0)
equation "d10 = ( 70.5 / 2 ) * 1 mm"
equation "d11 = ( 70.5 / 2 ) * 1 mm"
equation "d78 = ( ( 70.5 - 14 ) / 2 ) * 1 mm"
